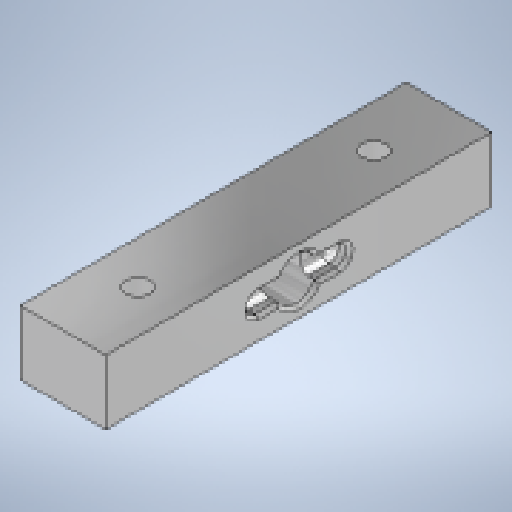
# Autodesk Inventor part: Rack - Top
Saved by Autodesk Inventor 2023.2 (Build 272271000, 271)
## iProperties
Created: 2024-01-12
Part Number: Rack - Top
Material: Aluminum 6061
Document SubType Name: Modeling
Designer: Nathan Cai
Density: 2.7 g/cm^3
Appearance: Aluminum - Flat
Mass: 16.8962 g
Surface Area: 31.6763 cm^2
Volume: 6.25786 cm^3
Author: Nathan Cai
Autodesk Inventor part; units mm, degrees
ref_plane "YZ Plane" through (0, 0, 0) normal (1, 0, 0) x (0, 1, 0)
ref_plane "XZ Plane" through (0, 0, 0) normal (0, 1, 0) x (-1, 0, 0)
ref_plane "XY Plane" through (0, 0, 0) normal (0, 0, 1) x (1, 0, 0)
sketch "Sketch1" plane through (0, 0, 0) normal (0, 1, 0) x (-1, 0, 0)
  line L0 (0, 17.4625) -> (0, 17.4625) construction
  line L1 (0, 17.4625) -> (0, -17.4625) construction
  line L2 (0, -17.4625) -> (0, -17.4625) construction
  line L3 (0, -17.4625) -> (0, 17.4625) construction
  line L4 (0, 17.4625) -> (0, -17.4625) construction
  line L5 (0, 17.4625) -> (0, -17.4625) construction
  circle A0 centre (0, 17.4625) radius 1.7526
  circle A1 centre (0, -17.4625) radius 1.7526
  circle A2 centre (0, 17.4625) radius 1.7526
  circle A3 centre (0, -17.4625) radius 1.7526
  line L6 (-6.35, 28.575) -> (6.35, 28.575)
  line L7 (6.35, 28.575) -> (6.35, -28.575)
  line L8 (6.35, -28.575) -> (-6.35, -28.575)
  line L9 (-6.35, -28.575) -> (-6.35, 28.575)
  line L10 (-6.35, 28.575) -> (6.35, -28.575) construction
  line L11 (6.35, 28.575) -> (-6.35, -28.575) construction
  line L12 (6.35, 28.575) -> (12.7, 28.575)
  line L13 (12.7, 28.575) -> (12.7, -28.575)
  line L14 (12.7, -28.575) -> (6.35, -28.575)
  line L15 (6.35, -28.575) -> (6.35, 28.575)
  line L16 (6.35, 12.7) -> (12.7, 19.05)
  line L17 (6.35, 0) -> (12.7, 0) construction
  line L18 (6.35, -12.7) -> (12.7, -19.05)
  point P0 (0, 0)
  point P1 (12.7, -19.05)
  dimension "d0" = 0
  dimension "d1" = 34.925
  dimension "d2" = 3.5052
  dimension "d5" = 34.925
  dimension "d8" = 0
  dimension "d11" = 12.7
  dimension "d12" = 57.15
  dimension "d40" = 6.35
  dimension "d41" = 9.525
  dimension "d42" = 12.7
  constraints: 38 end point, 6 equal length, 6 midpoint, 4 centre point, 4 horizontal, 3 coincident, 3 perpendicular, 3 point on line, 3 symmetric about line, 1 vertical, 5 other
  measures "d0" distance of L1.end L2.end
  measures "d1" distance of L0.end L1.end
  measures "d2" diameter of A0
  measures "d5" distance of A0.centre A1.centre
  measures "d8" distance of A0.centre A2.centre
  measures "d11" distance of L7.end L8.end
  measures "d12" distance of L6.end L7.end
  measures "d40" distance of L13.end L14.end
  measures "d41" distance from line of L12 point (12.7, 19.05)
  measures "d42" distance from line of L17 point (6.35, 12.7)
extrude "Extrusion1" add sketch "Sketch1" along normal blind 9.525 contours L6 L7 L8 L9 | L12 L13 L16 L7 | L7 L18 L13 L14
sketch "Sketch2" plane through (6.35, 0, 28.575) normal (1, 0, 0) x (0, 0, -1)
  line L0 (28.575, 0) -> (28.575, 9.525) construction
  line L1 (41.275, 9.525) -> (15.875, 9.525) projected
  circle A0 centre (28.575, 4.7625) radius 3.175
  line L2 (0, 0) -> (57.15, 0) projected
  point P0 (57.15, 9.525)
  point P1 (0, 9.525)
  point P2 (25.4, 0)
  point P3 (16.2434, 0)
  dimension "d15" = 6.35
  dimension "d16" = 4.7625
  constraints: 2 end point, 2 midpoint, 1 centre point
  measures "d15" diameter of A0
  measures "d16" distance from line of L2 A0.centre
extrude "Extrusion2" cut sketch "Sketch2" against normal through all
sketch "Sketch5" plane through (6.35, 0, 28.575) normal (1, 0, 0) x (0, 0, -1)
  line L0 (0, 0) -> (0, 9.525) projected
  line L1 (0, 4.7625) -> (57.15, 4.7625) construction
  line L2 (57.15, 0) -> (57.15, 9.525) projected
  line L3 (22.575, 4.7625) -> (34.575, 4.7625) construction
  line L4 (22.575, 3.2625) -> (34.575, 3.2625)
  line L5 (34.575, 6.2625) -> (22.575, 6.2625)
  arc A0 (22.575, 6.2625) -> (22.575, 3.2625) centre (22.575, 4.7625) ccw
  arc A1 (34.575, 3.2625) -> (34.575, 6.2625) centre (34.575, 4.7625) ccw
  point P0 (28.575, 0)
  point P1 (28.575, 4.7625)
  dimension "d29" = 3
  dimension "d30" = 12
  constraints: 10 end point, 4 midpoint, 4 point on circle, 4 tangent, 2 centre point, 1 parallel, 1 point on line
  measures "d29" diameter of A1
  measures "d30" distance of L3.start L3.end
extrude "Extrusion5" cut sketch "Sketch5" against normal blind 3
fillet "Fillet3" radius 1.5 6 edges at (3.35, 6.2625, 4.3992) (3.35, 3.2625, 4.3992) (3.35, 4.7625, 7.5) (3.35, 4.7625, -7.5) (3.35, 3.2625, -4.3992) (3.35, 6.2625, -4.3992)
chamfer "Chamfer1" distance 0.5 angle 45 8 edges at (6.35, 3.2625, -4.3992) (6.35, 4.7625, -7.5) (6.35, 6.2625, -4.3992) (6.35, 7.9375, 0) (6.35, 6.2625, 4.3992) (6.35, 4.7625, 7.5) (6.35, 3.2625, 4.3992) (6.35, 1.5875, 0)
fillet "Fillet4" radius 6.35 4 edges at (-6.35, 4.7625, 12.7) (-6.35, 4.7625, -12.7) (-12.7, 4.7625, 19.05) (-12.7, 4.7625, -19.05)
ref_plane "Work Plane1" through (6.35, 0, 0) normal (0, 0, -1) x (-1, 0, 0)
sketch "Sketch6" plane through (6.35, 0, -28.575) normal (0, 0, -1) x (-1, 0, 0)
  line L0 (0, 0) -> (0, 9.525) projected
  line L1 (0, 4.7625) -> (19.05, 4.7625) construction
  line L2 (19.05, 0) -> (19.05, 9.525) projected
  line L3 (4.7625, 4.7625) -> (14.2875, 4.7625) construction
  line L4 (4.7625, 2.3813) -> (14.2875, 2.3812)
  line L5 (14.2875, 7.1437) -> (4.7625, 7.1438)
  arc A0 (4.7625, 7.1438) -> (4.7625, 2.3813) centre (4.7625, 4.7625) ccw
  arc A1 (14.2875, 2.3812) -> (14.2875, 7.1437) centre (14.2875, 4.7625) ccw
  circle A2 centre (4.7625, 4.7625) radius 1.65
  circle A3 centre (14.2875, 4.7625) radius 1.65
  point P0 (6.35, 0)
  point P1 (9.525, 4.7625)
  dimension "d44" = 4.7625
  dimension "d45" = 4.7625
  dimension "d46" = 4.7625
  dimension "d47" = 3.3
  dimension "d48" = 3.3
  constraints: 10 end point, 4 centre point, 4 point on circle, 4 tangent, 3 midpoint, 2 coincident, 2 point on line, 1 parallel
  measures "d44" diameter of A1
  measures "d45" distance from line of L0 L3.start
  measures "d46" distance from line of L2 L3.end
  measures "d47" diameter of A2
  measures "d48" diameter of A3
extrude "Extrusion6" add sketch "Sketch6" along normal blind 6.35
mirror "Mirror1" about plane through (6.35, 0, 0) normal (0, 0, -1) of "Extrusion6"
equation "\"d5\" = d1"
equation "\"d45\" = d44"
equation "\"d46\" = d44"
body "Solid1"
